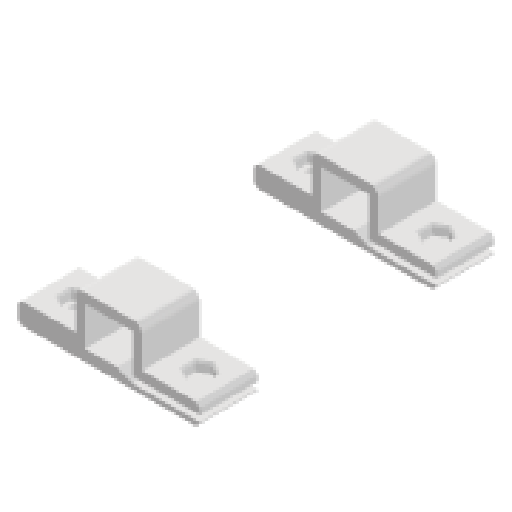
# Autodesk Inventor part: Motor Mount
Saved by Autodesk Inventor 2026.1 (Build 301233020, 233B)
## iProperties
Created: 2026-02-19
Part Number: Motor Mount
Material: Generic
Document SubType Name: Modeling
Designer: Snail
Density: 1 g/cm^3
Appearance: Default
Author: Snail
Autodesk Inventor part; units mm, degrees
ref_plane "YZ Plane" through (0, 0, 0) normal (1, 0, 0) x (0, 1, 0)
ref_plane "XZ Plane" through (0, 0, 0) normal (0, 1, 0) x (-1, 0, 0)
ref_plane "XY Plane" through (0, 0, 0) normal (0, 0, 1) x (1, 0, 0)
sketch "Sketch1" plane through (0, 0, 0) normal (0, 0, 1) x (1, 0, 0)
  line L0 (0, 0) -> (2.5, 0)
  line L1 (2.5, 0) -> (2.5, 10.15)
  line L2 (0, 12.65) -> (0, 0)
  line L3 (17.3, 12.65) -> (17.3, 10.15)
  line L4 (14.8, 10.15) -> (2.5, 10.15)
  line L5 (14.8, 10.15) -> (14.8, 0)
  line L6 (14.8, 0) -> (17.3, 0)
  line L7 (17.3, 0) -> (17.3, 10.15)
  line L8 (0, 12.65) -> (17.3, 12.65)
  line L9 (0, 0) -> (-15, 0)
  line L10 (-15, 0) -> (-15, 2.5)
  line L11 (-15, 2.5) -> (0, 2.5)
  line L12 (0, 2.5) -> (0, 0)
  line L13 (17.3, 0) -> (32.3, 0)
  line L14 (32.3, 0) -> (32.3, 2.5)
  line L15 (32.3, 2.5) -> (17.3, 2.5)
  line L16 (17.3, 2.5) -> (17.3, 0)
  point P0 (0, 2.5)
  point P1 (0, 2.5)
  dimension "d2" = 2.5
  dimension "d4" = 2.5
  dimension "d6" = 15
  dimension "d7" = 2.5
  dimension "d17" = 12.3
  dimension "d18" = 10.15
  constraints: 34 end point, 7 parallel, 4 horizontal, 3 equal length, 3 perpendicular, 2 point on line, 1 vertical alignment
  measures "d2" distance between parallel lines of L2 L1
  measures "d4" distance between parallel lines of L8 L4
  measures "d6" distance between parallel lines of L14 L16
  measures "d7" distance between parallel lines of L9 L11
  measures "d17" distance between parallel lines of L5 L1
  measures "d18" distance between parallel lines of L4 L9
extrude "Extrusion1" add sketch "Sketch1" along normal blind 15
sketch "Sketch3" plane through (0, 0, 0) normal (0, 0, -1) x (-1, 0, 0)
  line L0 (15, 0) -> (-2.5, 0) projected
  line L1 (15, 0) -> (-32.3, 0)
  line L2 (-32.3, 0) -> (-32.3, -3)
  line L3 (-32.3, -3) -> (15, -3)
  line L4 (15, -3) -> (15, 0)
  line L5 (-32.3, 0) -> (-14.8, 0)
  line L6 (-14.8, 0) -> (-14.8, -1.65)
  line L7 (-14.8, -1.65) -> (-32.3, -1.65)
  line L8 (-32.3, -1.65) -> (-32.3, 0)
  line L9 (-14.8, -1.65) -> (-10.8, 0)
  line L10 (-14.8, 10.15) -> (-14.8, 0) projected
  point P0 (0, 0)
  point P1 (-32.3, 2.5)
  dimension "d19" = 3
  dimension "d20" = 1.65
  dimension "d23" = 4
  constraints: 18 end point, 4 parallel, 2 horizontal, 2 perpendicular, 2 vertical alignment, 1 point on line
  measures "d19" distance between parallel lines of L0 L3
  measures "d20" distance between parallel lines of L1 L7
  measures "d23" distance from line of L9.end L10
extrude "Extrusion3" add sketch "Sketch3" against normal up to surface (15 mm away) contours L4 L3 L2 L7 L9 L1 L0
sketch "Sketch2" plane through (-15, 2.5, 0) normal (0, 1, 0) x (1, 0, 0)
  circle A0 centre (7.5, -7.5) radius 1.5
  circle A1 centre (39.8, -7.5) radius 1.5
  line L0 (15, 0) -> (0, 0) projected
  line L1 (0, 0) -> (0, -15) projected
  line L2 (17.5, 0) -> (29.8, 0) projected
  line L3 (23.65, 0) -> (23.65, -15)
  line L4 (17.5, -15) -> (29.8, -15) projected
  point P0 (7.5, 0)
  point P1 (0, -7.5)
  dimension "d10" = 3
  constraints: 4 midpoint, 2 centre point, 2 end point, 1 equal radius, 1 horizontal alignment, 1 vertical alignment, 1 other
  measures "d10" diameter of A0
extrude "Extrusion2" cut sketch "Sketch2" against normal up to surface (5.5 mm away)
sketch "Sketch4" plane through (-15, 2.5, 0) normal (0, 1, 0) x (1, 0, 0)
  line L0 (7.5, -4.2668) -> (10.3, -5.8834)
  line L1 (10.3, -5.8834) -> (10.3, -9.1166)
  line L2 (10.3, -9.1166) -> (7.5, -10.7332)
  line L3 (7.5, -10.7332) -> (4.7, -9.1166)
  line L4 (4.7, -9.1166) -> (4.7, -5.8834)
  line L5 (4.7, -5.8834) -> (7.5, -4.2668)
  line L6 (42.6, -5.8834) -> (42.6, -9.1166)
  line L7 (42.6, -9.1166) -> (39.8, -10.7332)
  line L8 (39.8, -10.7332) -> (37, -9.1166)
  line L9 (37, -9.1166) -> (37, -5.8834)
  line L10 (37, -5.8834) -> (39.8, -4.2668)
  line L11 (39.8, -4.2668) -> (42.6, -5.8834)
  circle A0 centre (39.8, -7.5) radius 1.5 projected
  circle A1 centre (7.5, -7.5) radius 1.5 projected
  line L12 (47.3, 0) -> (0, 0) projected
  line L13 (23.65, 0) -> (23.65, -15)
  line L14 (47.3, -15) -> (0, -15) projected
  point P0 (15, 0)
  point P1 (39.8, -7.5)
  dimension "d28" = 5.6
  constraints: 26 end point, 2 coincident, 2 midpoint, 1 symmetric about line, 1 vertical alignment, 28 other
  measures "d28" distance between parallel lines of L1 L4
extrude "Extrusion4" cut sketch "Sketch4" against normal up to surface (2.5 mm away)
chamfer "Chamfer3" distance 0.5 angle 45 15 edges at (26.2, 2.5, 9.9249) (23.4, 2.5, 9.9249) (22, 2.5, 7.5) (23.4, 2.5, 5.0751) (26.2, 2.5, 5.0751) (27.6, 2.5, 7.5) (-6.1, 2.5, 5.0751) (-4.7, 2.5, 7.5) (-6.1, 2.5, 9.9249) (-8.9, 2.5, 9.9249) (-10.3, 2.5, 7.5) (-8.9, 2.5, 5.0751) (-9, -3, 7.5) (23.3, -3, 7.5) (23.3, -1.65, 7.5)
fillet "Fillet2" radius 2 2 edges at (17.3, 12.65, 7.5) (0, 12.65, 7.5)
chamfer "Chamfer4" distance 1 angle 45 4 edges at (-15, -3, 7.5) (32.3, -3, 7.5) (32.3, 2.5, 7.5) (-15, 2.5, 7.5)
pattern_linear "Rectangular Pattern1" count 2 spacing 61.352 along (0, 0, 1) of "Extrusion1", "Extrusion3", "Extrusion2", "Extrusion4", "Chamfer3", "Fillet2", "Chamfer4"
equation "\"d2\" = Thick"
equation "\"d4\" = Thick"
equation "\"d7\" = Thick"
equation "\"d8\" = d6"
equation "\"Thick\" = 2.5"
equation "\"width\" = 12"
body "Solid1"
